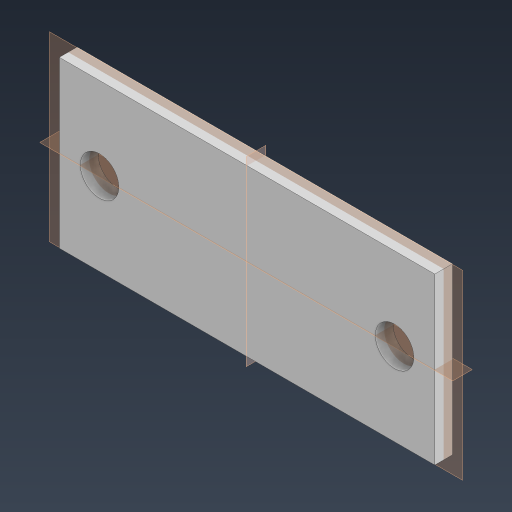
# Autodesk Inventor part: Фиксатор
Saved by Autodesk Inventor 2023.2 (Build 272271030, 271C)
## iProperties
Created: 2026-01-05
Part Number: Фиксатор
Material: Типовые
Document SubType Name: Modeling
Designer: Олег Коноваленко
Density: 1 g/cm^3
Appearance: По умолчанию
Author: Олег Коноваленко
Autodesk Inventor part; units mm, degrees
sketch "Эскиз1" plane through (0, 0, 0) normal (0, 0, 1) x (1, 0, 0)
  line L0 (-21, -9.25) -> (21, -9.25)
  line L1 (21, -9.25) -> (21, 9.25)
  line L2 (21, 9.25) -> (-21, 9.25)
  line L3 (-21, 9.25) -> (-21, -9.25)
  line L4 (-21, -9.25) -> (21, 9.25) construction
  line L5 (21, -9.25) -> (-21, 9.25) construction
  point P0 (0, 0)
  dimension "d0" = 42
  dimension "d1" = 18.5
  constraints: 12 end point, 2 midpoint, 2 parallel, 1 horizontal, 1 perpendicular
  measures "d0" distance of L1.end L2.end
  measures "d1" distance of L0.end L1.end
extrude "Выдавливание1" add sketch "Эскиз1" along normal mid plane 2
sketch "Эскиз2" plane through (0, 0, 1) normal (0, 0, 1) x (1, 0, 0)
  circle A0 centre (-16.5, 0) radius 2.15 projected
  circle A1 centre (16.5, 0) radius 2.15 projected
  point P0 (0, 0)
extrude "Выдавливание2" cut sketch "Эскиз2" against normal up to next
